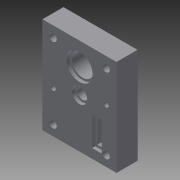
# Autodesk Inventor part: Guia
Saved by Autodesk Inventor 2015 (Build 190159000, 159)
## iProperties
Created: 2015-11-06
Part Number: Guia
Material: Generic
Document SubType Name: Modeling
Designer: EriveltonDell
Density: 1 g/cm^3
Appearance: Default
Author: EriveltonDell
Autodesk Inventor part; units mm, degrees
ref_plane "YZ Plane" through (0, 0, 0) normal (1, 0, 0) x (0, 1, 0)
ref_plane "XZ Plane" through (0, 0, 0) normal (0, 1, 0) x (-1, 0, 0)
ref_plane "XY Plane" through (0, 0, 0) normal (0, 0, 1) x (1, 0, 0)
sketch "Sketch1" plane through (0, 0, 0) normal (0, 1, 0) x (-1, 0, 0)
  circle A0 centre (0, 0) radius 10.5
  line L0 (0, 0) -> (0, -23.5)
  circle A1 centre (0, -23.5) radius 5.25
  line L1 (0, -23.5) -> (0, -35.25)
  line L2 (-14, -35.25) -> (-14, -58.75)
  line L3 (-14, -58.75) -> (-19, -58.75)
  line L4 (-19, -58.75) -> (-19, -35.25)
  line L5 (-35.25, 21.625) -> (35.25, 21.625)
  line L6 (-35.25, 21.625) -> (35.25, 21.625) construction
  line L7 (35.25, 21.625) -> (25.25, 21.625)
  line L8 (-35.25, 21.625) -> (35.25, 21.625)
  line L9 (35.25, 21.625) -> (35.25, -69.875)
  line L10 (35.25, -69.875) -> (-35.25, -69.875)
  line L11 (-35.25, -69.875) -> (-35.25, 21.625)
  line L12 (-35.25, 21.625) -> (-35.25, 11.625)
  line L13 (-35.25, 11.625) -> (-25.25, 11.625)
  circle A2 centre (-25.25, 11.625) radius 3.5
  line L14 (35.25, 21.625) -> (25.25, 21.625)
  line L15 (25.25, 21.625) -> (25.25, 11.625)
  circle A3 centre (25.25, 11.625) radius 3.5
  line L16 (35.25, -69.875) -> (25.25, -69.875)
  line L17 (25.25, -69.875) -> (25.25, -59.875)
  circle A4 centre (25.25, -59.875) radius 3.5
  line L18 (-35.25, -69.875) -> (-25.25, -69.875)
  line L19 (-25.25, -69.875) -> (-25.25, -59.875)
  circle A5 centre (-25.25, -59.875) radius 3.5
  line L20 (-25.25, 11.625) -> (-25.25, -18.375)
  line L21 (25.25, -59.875) -> (25.25, -29.875)
  circle A6 centre (-25.25, -18.375) radius 2.5
  circle A7 centre (25.25, -29.875) radius 2.5
  line L22 (-19, -35.25) -> (-14, -35.25)
  dimension "d0" = 21
  dimension "d1" = 23.5
  dimension "d2" = 10.5
  dimension "d3" = 11.75
  dimension "d5" = 23.5
  dimension "d6" = 5
  dimension "d7" = 23.5
  dimension "d9" = 70.5
  dimension "d40" = 21.625
  dimension "d41" = 70.5
  dimension "d42" = 91.5
  dimension "d43" = 10
  dimension "d44" = 10
  dimension "d45" = 7
  dimension "d46" = 10
  dimension "d47" = 10
  dimension "d48" = 90
  dimension "d50" = 7
  dimension "d51" = 10
  dimension "d52" = 10
  dimension "d53" = 7
  dimension "d54" = 10
  dimension "d55" = 10
  dimension "d56" = 7
  dimension "d60" = 30
  dimension "d61" = 30
  dimension "d62" = 5
  dimension "d63" = 5
  dimension "d64" = 14
  constraints: 46 end point, 8 centre point, 8 coincident, 6 perpendicular, 4 horizontal, 4 point on line, 4 vertical, 3 equal length, 1 collinear
  measures "d0" diameter of A0
  measures "d1" distance of L0.start L0.end
  measures "d2" diameter of A1
  measures "d3" distance of L1.start L1.end
  measures "d5" distance of L2.start L2.end
  measures "d6" distance of L2.end L3.end
  measures "d7" distance of L3.end L4.end
  measures "d9" distance of L5.start L5.end
  measures "d40" distance from line of L5 L0.start
  measures "d41" distance of L9.end L10.end
  measures "d42" distance of L8.end L9.end
  measures "d43" distance of L5.start L12.end
  measures "d44" distance of L12.end L13.end
  measures "d45" diameter of A2
  measures "d46" distance of L8.end L7.end
  measures "d47" distance of L7.end L15.end
  measures "d48" angle of L15 L14
  measures "d50" diameter of A3
  measures "d51" distance of L9.end L16.end
  measures "d52" distance of L16.end L17.end
  measures "d53" diameter of A4
  measures "d54" distance of L10.end L18.end
  measures "d55" distance of L18.end L19.end
  measures "d56" diameter of A5
  measures "d60" distance of L20.start L20.end
  measures "d61" distance of L21.start L21.end
  measures "d62" diameter of A6
  measures "d63" diameter of A7
  measures "d64" distance between parallel lines of L2 L1
extrude "Extrusion1" add sketch "Sketch1" along normal blind 20
hole "Hole1" at (0, 0, 0) direction (0, 1, 0) diameter 3 end through all counterbore diameter 25 counterbore depth 3
hole "Hole2" at (0, 0, -23.5) direction (0, 1, 0) diameter 3 end through all counterbore diameter 14.5 counterbore depth 3
sketch "Sketch2" plane through (0, 0, 0) normal (0, -1, 0) x (1, 0, 0)
  line L0 (12, -33.25) -> (21, -33.25)
  line L1 (21, -33.25) -> (21, -61)
  line L2 (21, -61) -> (12, -61)
  line L3 (12, -61) -> (12, -33.25)
  point P0 (0, 0)
  dimension "d85" = 33.25
  dimension "d86" = 12
  dimension "d87" = 9
  dimension "d88" = 27.75
  constraints: 8 end point, 2 parallel, 1 horizontal, 1 perpendicular
  measures "d85" distance from line of L0 point (0, 0)
  measures "d86" distance from line of L3 point (0, 0)
  measures "d87" distance of L0.start L0.end
  measures "d88" distance of L0.end L1.end
extrude "Extrusion2" cut sketch "Sketch2" against normal blind 3
body "Solid1"
